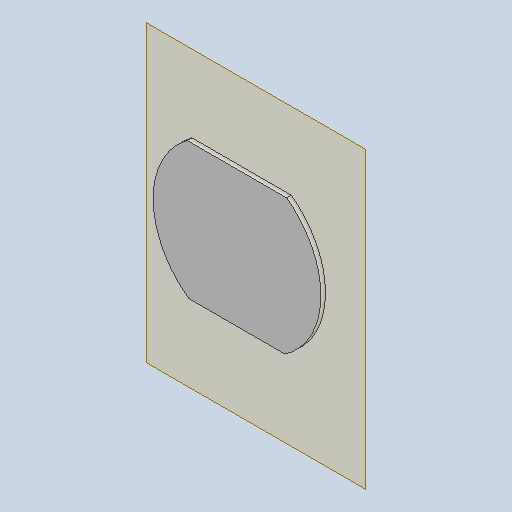
# Autodesk Inventor part: талия
Saved by Autodesk Inventor 2023.1 (Build 271208000, 208)
## iProperties
Created: 2025-01-17
Part Number: талия
Material: Типовые
Document SubType Name: Modeling
Designer: DELL
Density: 1 g/cm^3
Appearance: По умолчанию
Author: DELL
Autodesk Inventor part; units mm, degrees
ref_plane "YZ Plane" through (0, 0, 0) normal (1, 0, 0) x (0, 1, 0)
ref_plane "XZ Plane" through (0, 0, 0) normal (0, 1, 0) x (-1, 0, 0)
ref_plane "XY Plane" through (0, 0, 0) normal (0, 0, 1) x (1, 0, 0)
ref_plane "РабПлоскость1" through (-0.0725, -0.4347, 0) normal (0, 0, 1) x (1, 0, 0)
sketch "Эскиз1" plane through (-0.0725, -0.4347, 0) normal (0, 0, 1) x (1, 0, 0)
  line L0 (-1.9997, -72.1072) -> (-1.9997, 72.1074) construction
  line L1 (-1.9997, 72.1074) -> (0, 72.1074) construction
  line L2 (2.0003, 72.1074) -> (2.0003, -72.1072) construction
  line L3 (2.0003, -72.1072) -> (-1.9997, -72.1072) construction
  line L4 (48.0003, 58.8035) -> (-47.9997, 58.8035) construction
  line L5 (-47.9997, 58.8035) -> (-47.9997, 62.8035) construction
  line L6 (-47.9997, 62.8035) -> (48.0003, 62.8035) construction
  line L7 (48.0003, 62.8035) -> (48.0003, 58.8035) construction
  line L8 (-47.9997, -58.9592) -> (48.0003, -58.9592) construction
  line L9 (48.0003, -58.9592) -> (48.0003, -62.9592) construction
  line L10 (48.0003, -62.9592) -> (-47.9997, -62.9592) construction
  line L11 (-47.9997, -62.9592) -> (-47.9997, -58.9592) construction
  line L12 (-42.9694, 58.8035) -> (42.9958, 58.8035)
  line L13 (-41.5432, -58.9592) -> (41.5655, -58.9592)
  arc A0 (2.0003, 72.0815) -> (0, 72.1074) centre (0.0725, 0.4347) ccw
  arc A1 (-36.9363, 62.8035) -> (-35.1512, -62.9592) centre (0.0725, 0.4347) ccw
  arc A2 (-1.9997, -72.0756) -> (2.0003, -72.0796) centre (0.0725, 0.4347) ccw
  arc A3 (35.1512, -62.9592) -> (36.9433, 62.8035) centre (0.0725, 0.4347) ccw
  constraints: 28 end point, 12 point on circle, 11 point on line, 6 horizontal, 6 vertical, 4 centre point, 1 coincident, 12 other
extrude "Выдавливание1" add sketch "Эскиз1" along normal mid plane 4
